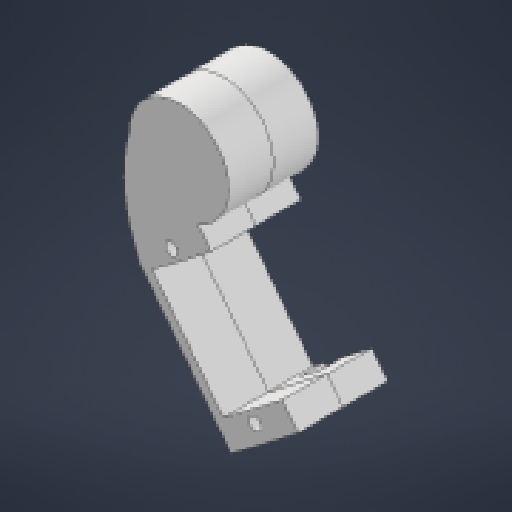
# Autodesk Inventor part: base
Saved by Autodesk Inventor 2026.1 (Build 301233020, 233B)
## iProperties
Created: 2025-11-20
Part Number: base
Material: 일반
Document SubType Name: Modeling
Designer: jaewook
Density: 1 g/cm^3
Appearance: 기본값
Author: jaewook
Autodesk Inventor part; units mm, degrees
ref_plane "YZ Plane" through (0, 0, 0) normal (1, 0, 0) x (0, 1, 0)
ref_plane "XZ Plane" through (0, 0, 0) normal (0, 1, 0) x (-1, 0, 0)
ref_plane "XY Plane" through (0, 0, 0) normal (0, 0, 1) x (1, 0, 0)
sketch "스케치2" plane through (0, 0, 0) normal (0, 0, 1) x (1, 0, 0)
  line L0 (168.2265, -29.7181) -> (182.0227, -47.7445)
  line L1 (191.5521, -40.4514) -> (177.7559, -22.4249)
  line L2 (177.7559, -22.4249) -> (168.2265, -29.7181)
  line L3 (172.1391, -30.8815) -> (212.5451, -83.6769) projected
  line L4 (175.1246, -38.7313) -> (184.654, -31.4381) construction
  line L5 (172.9912, -26.0715) -> (186.7874, -44.098) construction
  line L6 (185.1992, -45.3135) -> (187.5087, -48.3311)
  line L7 (187.5087, -48.3311) -> (190.6852, -45.9001)
  line L8 (190.6852, -45.9001) -> (188.3757, -42.8824)
  line L9 (176.3073, -16.4187) -> (196.9713, -43.4187)
  line L10 (196.9713, -43.4187) -> (183.4713, -53.7507)
  line L11 (183.4713, -53.7507) -> (162.8073, -26.7507)
  line L12 (162.8073, -26.7507) -> (176.3073, -16.4187)
  line L13 (176.3073, -16.4187) -> (183.4713, -53.7507) construction
  line L14 (196.9713, -43.4187) -> (162.8073, -26.7507) construction
  line L15 (182.0227, -47.7445) -> (185.1992, -45.3135)
  line L16 (188.3757, -42.8824) -> (191.5521, -40.4514)
  line L17 (177.8304, -21.8642) -> (192.1129, -40.5259)
  line L18 (192.1129, -40.5259) -> (188.9364, -42.957)
  line L19 (188.9364, -42.957) -> (191.2459, -45.9746)
  line L20 (191.2459, -45.9746) -> (187.4341, -48.8919)
  line L21 (187.4341, -48.8919) -> (185.1246, -45.8742)
  line L22 (185.1246, -45.8742) -> (181.9482, -48.3053)
  line L23 (181.9482, -48.3053) -> (167.6657, -29.6435)
  line L24 (167.6657, -29.6435) -> (177.8304, -21.8642)
  circle A0 centre (173, -8) radius 10 projected
  line L25 (185.1246, -45.8742) -> (188.9364, -42.957)
  circle A1 centre (171.4718, -24.0862) radius 1.25
  circle A2 centre (188.3068, -46.0833) radius 1.25
  arc A3 (163, -8.0077) -> (165.2941, -30) centre (193.8521, -15.9052) ccw
  point P0 (0, 0)
  point P1 (179.8893, -35.0847)
  point P2 (179.8893, -35.0847)
  point P3 (176.9087, -17.2045)
  point P4 (174.3632, -17.9067)
  point P5 (163.6763, -26.0857)
  dimension "d0" = 22.7
  dimension "d1" = 12
  dimension "d2" = 4
  dimension "d3" = 26.5
  dimension "d4" = 34
  dimension "d5" = 17
  dimension "d6" = 0.4
  dimension "d9" = 2.5
  dimension "d10" = 2.5
  dimension "d16" = 3.6
  constraints: 50 end point, 17 perpendicular, 10 parallel, 8 midpoint, 3 centre point, 2 point on circle, 2 point on line, 1 symmetric about line, 11 other
  measures "d0" distance of L1.start L1.end
  measures "d1" distance of L0.end L1.start
  measures "d2" distance of L6.end L7.end
  measures "d3" distance between parallel lines of L2 L7
  measures "d4" distance of L10.end L11.end
  measures "d5" distance of L9.end L10.end
  measures "d6" distance between parallel lines of L1 L17
  measures "d9" distance from line of L2 A1.centre
  measures "d10" diameter of A1
  measures "d16" distance from line of L3 point (179.889, -35.085)
extrude "돌출1" add sketch "스케치2" along normal mid plane 18 contours L25 L6 L7 L8 L19 L20 L21 | L25 L8 L7 L6 | L12 A0 L9 | L9 A0 L12 | L9 L10 L11 A3 L12 A0 | L12 A3 A0
sketch "스케치3" plane through (192.1129, -40.5259, -9) normal (-0.7941176, -0.6077641, 0) x (0, 0, 1)
  line L0 (18, 0) -> (0, 0) projected
  line L1 (18, 23.5) -> (18, 0) projected
  line L2 (0, 23.5) -> (18, 23.5) projected
  line L3 (0, 0) -> (0, 23.5) projected
  point P0 (9, 148.9416)
extrude "돌출2" cut sketch "스케치3" against normal blind 18
sketch "스케치4" plane through (196.9713, -43.4187, -9) normal (0.6077641, -0.7941176, 0) x (0.7941176, 0.6077641, 0)
  line L0 (0, 0) -> (-17, 0) projected
  line L1 (-12, 0) -> (-7, 0)
  line L2 (-7, 0) -> (-7, 5)
  line L3 (-7, 5) -> (-12, 5)
  line L4 (-12, 5) -> (-12, 0)
  point P0 (-130.03, 9)
  point P1 (-7, 0)
  constraints: 8 end point, 2 parallel, 1 horizontal, 1 perpendicular, 1 point on line
extrude "돌출3" cut sketch "스케치4" against normal blind 18
split body "분할1" result two bodies by plane through (0, 0, 0) normal (0, 0, 1) first body at (174.2785, -9.3972, 8.5)
